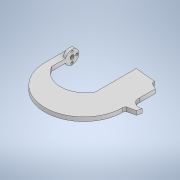
# Autodesk Inventor part: carma
Saved by Autodesk Inventor 2021 (Build 250183000, 183)
## iProperties
Created: 2021-03-22
Part Number: carma
Material: Generic
Document SubType Name: Modeling
Designer: Miss Oana
Density: 1 g/cm^3
Appearance: Default
Author: Miss Oana
Autodesk Inventor part; units mm, degrees
ref_plane "YZ Plane" through (0, 0, 0) normal (1, 0, 0) x (0, 1, 0)
ref_plane "XZ Plane" through (0, 0, 0) normal (0, 1, 0) x (-1, 0, 0)
ref_plane "XY Plane" through (0, 0, 0) normal (0, 0, 1) x (1, 0, 0)
sketch "prindere" plane through (0, 0, 0) normal (0, 0, 1) x (1, 0, 0)
  circle A0 centre (0, 0) radius 10 construction
  circle A1 centre (0, -7.1) radius 1.75 construction
  circle A2 centre (0, 7.1) radius 1.75 construction
  circle A3 centre (-7.1, 0) radius 1.75 construction
  circle A4 centre (7.1, 0) radius 1.75 construction
  circle A5 centre (0, 0) radius 1.65 construction
  dimension "d1" = 10
sketch "Sketch1" plane through (0, 0, 0) normal (0, 1, 0) x (-1, 0, 0)
  line L0 (67.0192, 27.1113) -> (57.0192, 27.1113) construction
  line L1 (57.0192, 27.1113) -> (57.0192, -7.8887)
  line L2 (57.0192, -7.8887) -> (67.0192, -7.8887)
  line L3 (67.0192, -7.8887) -> (67.0192, 27.1113)
  line L4 (-7.9808, 27.1113) -> (-47.9808, 27.1113) construction
  line L5 (-47.9808, 27.1113) -> (-47.9808, -20.8435)
  line L6 (-47.9808, -32.8887) -> (-7.9808, -32.8887) construction
  line L7 (-7.9808, -32.8887) -> (-7.9808, 27.1113)
  arc A0 (57.0192, 27.1113) -> (-7.9808, 27.1113) centre (24.5192, 9.6227) ccw
  arc A1 (67.0192, 27.1113) -> (-47.9808, 27.1113) centre (9.5192, 27.1113) ccw
  arc A2 (-50.0815, 23.591) -> (-47.9808, 27.1113) centre (-51.9808, 27.1113) ccw
  line L8 (-50.0815, 23.591) -> (-61.765, 20.853)
  line L9 (-61.765, 20.853) -> (-63.6478, 14.111)
  arc A3 (-47.9808, 2.187) -> (-63.6478, 14.111) centre (-59.4808, 3.3315) ccw
  line L10 (-7.9808, -32.8887) -> (-37.8292, -29.876)
  line L11 (-37.8292, -29.876) -> (-38.3378, -25.7069)
  line L12 (-38.3378, -25.7069) -> (-47.9808, -20.8435)
  line L13 (-47.9808, -20.8435) -> (-47.9808, -32.8887) construction
  point P0 (0, 0)
  dimension "d0" = 35
  dimension "d1" = 10
  dimension "d2" = 60
  dimension "d3" = 40
  dimension "d4" = 65
  dimension "d5" = 36.9066
  dimension "d6" = 12
  dimension "d7" = 4
  dimension "d8" = 7
  dimension "d9" = 11.5
  dimension "d10" = 30
  dimension "d11" = 10.8
  dimension "d12" = 4.2
  dimension "d13" = 11.5568
  dimension "d14" = 84.237
  dimension "d15" = 6.957
  dimension "d16" = 76.811
  dimension "d17" = 15.603
  dimension "d18" = 67.0192
  dimension "d19" = 7.8887
  dimension "d20" = 34.3956
  constraints: 28 end point, 8 point on circle, 5 parallel, 4 centre point, 3 perpendicular, 2 horizontal, 2 tangent, 1 collinear, 1 point on line
  measures "d0" distance of L2.end L0.start
  measures "d1" distance of L0.start L0.end
  measures "d2" distance of L6.end L4.start
  measures "d3" distance of L6.start L6.end
  measures "d4" distance between parallel lines of L7 L1
  measures "d5" radius of A0
  measures "d6" distance of L8.start L8.end
  measures "d7" distance of L4.end A2.centre
  measures "d8" distance of L8.end L9.end
  measures "d9" horizontal distance of A3.centre A3.start
  measures "d10" distance of L6.end L10.end
  measures "d11" distance of L11.end L5.end
  measures "d12" distance of L10.end L11.end
  measures "d13" radius of A3
  measures "d14" angle of L3 L10
  measures "d15" angle of L3 L11
  measures "d16" angle of L3 L8
  measures "d17" angle of L3 L9
  measures "d18" distance from line of point (0, 0) L3
  measures "d19" distance from line of point (0, 0) L2
  measures "d20" distance from line of point (0, 0) L8
extrude "Extrusion1" add sketch "Sketch1" along normal blind 6 contours A0 L7 L10 L11 L12 L5 A3 A1 L3 L2 L1 | L5 A3 L9 L8 A2
sketch "Sketch2" plane through (-57.0192, 0, 27.1113) normal (1, 0, 0) x (0, 0, -1)
  line L0 (0, 0) -> (35, 0) construction
  line L1 (35, 0) -> (35, 6) construction
  line L2 (0, 6) -> (35, 6) construction
  line L3 (0, 0) -> (0, 6) construction
  line L4 (0, 0) -> (0, 6) construction
  line L5 (0, 3) -> (35, 3) construction
  circle A0 centre (30, 3) radius 10
  circle A1 centre (30, 10.1) radius 1.75
  circle A2 centre (37.1, 3) radius 1.75
  circle A3 centre (30, -4.1) radius 1.75
  circle A4 centre (30, 3) radius 1.65
  point P0 (27.1113, 0)
  dimension "d23" = 5
  constraints: 5 centre point, 2 end point, 2 horizontal, 2 midpoint, 1 coincident, 9 other
extrude "Extrusion2" add sketch "Sketch2" against normal blind 4
sketch "Sketch3" plane through (-57.0192, 0, 27.1113) normal (1, 0, 0) x (0, 0, -1)
  arc A0 (20.4606, 0) -> (20.4606, 6) centre (30, 3) ccw projected
  circle A1 centre (30, 3) radius 3
  point P0 (27.1113, 0)
  dimension "d26" = 6
  constraints: 1 centre point, 1 coincident
  measures "d26" diameter of A1
extrude "Extrusion3" cut sketch "Sketch3" against normal through all
equation "\"d1\" = hmic"
equation "\"d0\" = lmic"
equation "\"d2\" = lmare"
equation "\"d3\" = hmare"
equation "\"d4\" = rcerc"
equation "\"d6\" = laripa"
equation "\"d7\" = rcerculet1"
equation "\"d8\" = haripa"
equation "\"d9\" = rcerculet2"
equation "\"d10\" = 0.5 * lmare"
equation "\"d11\" = 0.18 * lmare"
equation "\"d12\" = 0.07 * lmare"
equation "\"d21\" = grosime"
equation "\"lmic\" = 35"
equation "\"hmic\" = 10"
equation "\"rcerc\" = 65"
equation "\"lmare\" = 60"
equation "\"hmare\" = 40"
equation "\"rcerculet1\" = 4"
equation "\"rcerculet2\" = 11.5"
equation "\"laripa\" = 12"
equation "\"haripa\" = 7"
equation "\"grosime\" = 6"
body "Solid1"
